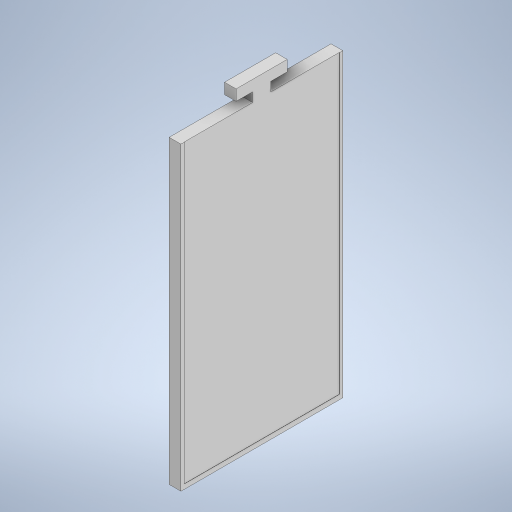
# Autodesk Inventor part: baseplateproto1
Saved by Autodesk Inventor 2023 (Build 270158000, 158)
## iProperties
Created: 2025-08-30
Part Number: baseplateproto1
Material: Generic
Document SubType Name: Modeling
Designer: ptato_qo49uko
Density: 1 g/cm^3
Appearance: Default
Author: ptato_qo49uko
Autodesk Inventor part; units mm, degrees
ref_plane "YZ Plane" through (0, 0, 0) normal (1, 0, 0) x (0, 1, 0)
ref_plane "XZ Plane" through (0, 0, 0) normal (0, 1, 0) x (-1, 0, 0)
ref_plane "XY Plane" through (0, 0, 0) normal (0, 0, 1) x (1, 0, 0)
sketch "Sketch1" plane through (0, 0, 0) normal (1, 0, 0) x (0, 1, 0)
  line L0 (82.3549, 41.969) -> (-47.6451, 41.969)
  line L1 (-47.6451, 41.969) -> (-47.6451, -28.031)
  line L2 (-47.6451, -28.031) -> (82.3549, -28.031)
  line L3 (82.3549, -28.031) -> (82.3549, 41.969)
  point P0 (0, 0)
  dimension "d0" = 130
  dimension "d1" = 70
  constraints: 8 end point, 2 parallel, 1 horizontal, 1 perpendicular
  measures "d0" distance of L2.end L1.end
  measures "d1" distance of L1.end L0.end
extrude "Extrusion1" add sketch "Sketch1" along normal blind 5
sketch "Sketch13" plane through (5, 0, 0) normal (1, 0, 0) x (0, 0, -1)
  line L0 (-41.969, -47.6451) -> (28.031, -47.6451) projected
  line L1 (28.031, 82.3549) -> (-41.969, 82.3549) projected
  line L2 (28.031, -47.6451) -> (26.531, -47.6451)
  line L3 (26.531, -47.6451) -> (26.531, 82.3549)
  line L4 (26.531, 82.3549) -> (28.031, 82.3549)
  line L5 (28.031, 82.3549) -> (28.031, -47.6451)
  line L6 (-41.969, 82.3549) -> (-41.969, -47.6451) projected
  line L7 (28.031, 82.3549) -> (-41.969, 82.3549) projected
  line L8 (-41.969, -47.6451) -> (-40.469, -47.6451)
  line L9 (-40.469, -47.6451) -> (-40.469, 82.3549)
  line L10 (-40.469, 82.3549) -> (-41.969, 82.3549)
  line L11 (-41.969, 82.3549) -> (-41.969, -47.6451)
  line L12 (28.031, -47.6451) -> (-41.969, -47.6451)
  line L13 (-41.969, -47.6451) -> (-41.969, -45.6451)
  line L14 (-41.969, -45.6451) -> (28.031, -45.6451)
  line L15 (28.031, -45.6451) -> (28.031, -47.6451)
  point P0 (0, 0)
  point P1 (10.031, 62.3549)
  point P2 (-5.969, 62.3549)
  point P3 (26.531, -45.6451)
  point P4 (-40.469, -45.6451)
  point P5 (18.031, 62.3549)
  dimension "d42" = 1.5
  dimension "d43" = 1.5
  dimension "d44" = 2
  constraints: 24 end point, 6 parallel, 3 horizontal, 3 perpendicular, 1 point on line, 4 other
  measures "d42" distance of L3.end L4.end
  measures "d43" distance of L10.end L9.end
  measures "d44" distance of L12.end L13.end
extrude "Extrusion7" add sketch "Sketch13" along normal blind 0.1 contours L6 L14 L9 L0 | L9 L14 L3 L0 | L6 L1 L9 L14 | L3 L14 L5 L0 | L3 L1 L5 L14
sketch "Sketch14" plane through (0, 82.3549, 41.969) normal (0, 1, 0) x (1, 0, 0)
  line L0 (5, 1.5) -> (5, 68.5) projected
  line L1 (5, 68.5) -> (5, 46.05)
  line L2 (5, 1.5) -> (5, 23.95)
  line L3 (5, 46.05) -> (0, 46.05)
  line L4 (5, 29.05) -> (5, 46.05)
  line L5 (0, 70) -> (0, 0) projected
  line L6 (5, 46.05) -> (0, 46.05)
  line L7 (0, 46.05) -> (0, 23.95)
  line L8 (0, 23.95) -> (5, 23.95)
  line L9 (5, 23.95) -> (5, 46.05)
  point P0 (0, 41.969)
  dimension "d47" = 22.45
  dimension "d48" = 22.45
  constraints: 16 end point, 3 point on line, 2 horizontal, 2 parallel, 1 perpendicular
  measures "d47" distance of L0.end L1.end
  measures "d48" distance of L0.start L2.end
extrude "Extrusion8" add sketch "Sketch14" along normal blind 8.65
sketch "Sketch15" plane through (5, 0, 0) normal (1, 0, 0) x (0, 0, -1)
  line L0 (28.031, 82.3549) -> (4.081, 82.3549) projected
  line L1 (4.081, 82.3549) -> (-3.069, 82.3549)
  line L2 (-3.069, 82.3549) -> (-3.069, 86.3549)
  line L3 (-3.069, 86.3549) -> (4.081, 86.3549)
  line L4 (4.081, 86.3549) -> (4.081, 82.3549)
  line L5 (-18.019, 82.3549) -> (-40.469, 82.3549) projected
  line L6 (-18.019, 82.3549) -> (-10.869, 82.3549)
  line L7 (-10.869, 82.3549) -> (-10.869, 86.3549)
  line L8 (-10.869, 86.3549) -> (-18.019, 86.3549)
  line L9 (-18.019, 86.3549) -> (-18.019, 82.3549)
  point P0 (0, 0)
  dimension "d51" = 7.15
  dimension "d52" = 7.15
  dimension "d55" = 4
  constraints: 16 end point, 4 parallel, 2 horizontal, 2 perpendicular, 1 point on line
  measures "d51" distance of L2.end L3.end
  measures "d52" distance of L8.end L7.end
  measures "d55" distance of L6.end L7.end
extrude "Extrusion9" cut sketch "Sketch15" against normal blind 8.65
body "Solid1"
